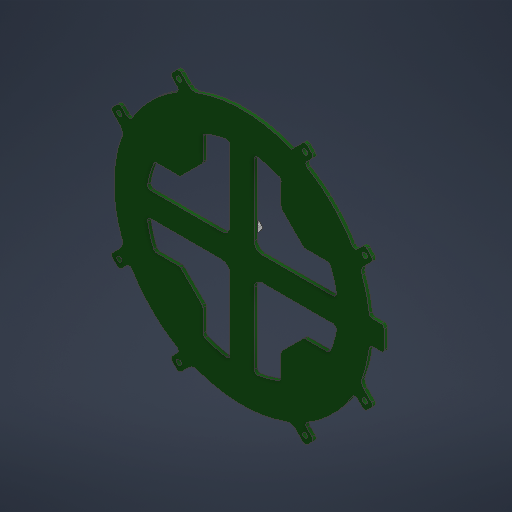
# Autodesk Inventor part: Line Board
Saved by Autodesk Inventor 2026.1 (Build 301233020, 233B)
## iProperties
Created: 2025-11-07
Part Number: Line Board
Material: Generic
Document SubType Name: Modeling
Designer: Bahaa
Density: 1 g/cm^3
Appearance: Default
Author: Bahaa
Autodesk Inventor part; units mm, degrees
ref_plane "YZ Plane" through (0, 0, 0) normal (1, 0, 0) x (0, 1, 0)
ref_plane "XZ Plane" through (0, 0, 0) normal (0, 1, 0) x (-1, 0, 0)
ref_plane "XY Plane" through (0, 0, 0) normal (0, 0, 1) x (1, 0, 0)
sketch "Sketch1" plane through (0, 0, 0) normal (0, 1, 0) x (-1, 0, 0)
  circle A0 centre (0, 0) radius 79
  circle A1 centre (0, 0) radius 59
  line L0 (-75, 7.5) -> (75, 7.5)
  line L1 (75, 7.5) -> (75, -7.5)
  line L2 (75, -7.5) -> (-75, -7.5)
  line L3 (-75, -7.5) -> (-75, 7.5)
  line L4 (-75, 7.5) -> (75, -7.5) construction
  line L5 (75, 7.5) -> (-75, -7.5) construction
  line L6 (-7.5, -75) -> (-7.5, 75)
  line L7 (7.5, 75) -> (7.5, -75)
  line L8 (75, -7.5) -> (-75, -7.5)
  line L9 (-75, 7.5) -> (75, 7.5)
  line L10 (7.5, 75) -> (7.5, -75)
  line L11 (-7.5, -75) -> (-7.5, 75)
  line L12 (7.5, 25) -> (-7.5, 25)
  line L13 (-25, 7.5) -> (-25, -7.5)
  line L14 (-7.5, -25) -> (7.5, -25)
  line L15 (25, -7.5) -> (25, 7.5)
  line L16 (25, 25) -> (-25, -25) construction
  line L17 (-25, 25) -> (25, -25) construction
  line L18 (-7.5, 25) -> (-25, 7.5)
  line L19 (25, 7.5) -> (7.5, 25)
  line L20 (25, -7.5) -> (7.5, -25)
  line L21 (-25, -7.5) -> (-7.5, -25)
  line L22 (0, 0) -> (57.2756, -57.2756) construction
  line L23 (57.2756, -57.2756) -> (38.8909, -75.6604) construction
  circle A2 centre (38.8909, -75.6604) radius 1.6
  line L24 (38.8909, -75.6604) -> (41.7193, -72.832) construction
  line L25 (41.7193, -72.832) -> (44.5477, -75.6604)
  line L26 (44.5477, -75.6604) -> (38.8909, -70.0036)
  line L27 (38.8909, -70.0036) -> (33.234, -75.6604) construction
  line L28 (33.234, -75.6604) -> (38.8909, -81.3173)
  line L29 (38.8909, -81.3173) -> (44.5477, -75.6604)
  line L30 (33.234, -75.6604) -> (30.4637, -72.8901)
  line L31 (38.8909, -70.0036) -> (38.0953, -69.208)
  circle A3 centre (75.6604, -38.8909) radius 1.6
  line L32 (75.6604, -38.8909) -> (72.832, -41.7193) construction
  line L33 (72.832, -41.7193) -> (75.6604, -44.5477)
  line L34 (75.6604, -44.5477) -> (70.0036, -38.8909)
  line L35 (70.0036, -38.8909) -> (75.6604, -33.234) construction
  line L36 (75.6604, -33.234) -> (81.3173, -38.8909)
  line L37 (81.3173, -38.8909) -> (75.6604, -44.5477)
  line L38 (75.6604, -33.234) -> (72.8901, -30.4637)
  line L39 (70.0036, -38.8909) -> (69.208, -38.0953)
  line L40 (70.0036, 38.8909) -> (69.208, 38.0953)
  line L41 (75.6604, 33.234) -> (72.8901, 30.4637)
  line L42 (70.0036, 38.8909) -> (75.6604, 33.234) construction
  line L43 (75.6604, 38.8909) -> (72.832, 41.7193) construction
  circle A4 centre (75.6604, 38.8909) radius 1.6
  line L44 (75.6604, 44.5477) -> (70.0036, 38.8909)
  line L45 (75.6604, 33.234) -> (81.3173, 38.8909)
  line L46 (81.3173, 38.8909) -> (75.6604, 44.5477)
  line L47 (57.2756, 57.2756) -> (75.6604, 38.8909) construction
  line L48 (72.832, 41.7193) -> (75.6604, 44.5477)
  line L49 (38.8909, 70.0036) -> (38.0953, 69.208)
  line L50 (41.7193, 72.832) -> (44.5477, 75.6604)
  line L51 (44.5477, 75.6604) -> (38.8909, 70.0036)
  line L52 (38.8909, 75.6604) -> (41.7193, 72.832) construction
  circle A5 centre (38.8909, 75.6604) radius 1.6
  line L53 (38.8909, 81.3173) -> (44.5477, 75.6604)
  line L54 (38.8909, 70.0036) -> (33.234, 75.6604) construction
  line L55 (33.234, 75.6604) -> (30.4637, 72.8901)
  line L56 (33.234, 75.6604) -> (38.8909, 81.3173)
  line L57 (-38.8909, 70.0036) -> (-38.0953, 69.208)
  line L58 (-33.234, 75.6604) -> (-30.4637, 72.8901)
  line L59 (-38.8909, 70.0036) -> (-33.234, 75.6604) construction
  line L60 (-38.8909, 75.6604) -> (-41.7193, 72.832) construction
  circle A6 centre (-38.8909, 75.6604) radius 1.6
  line L61 (-44.5477, 75.6604) -> (-38.8909, 70.0036)
  line L62 (-33.234, 75.6604) -> (-38.8909, 81.3173)
  line L63 (-38.8909, 81.3173) -> (-44.5477, 75.6604)
  line L64 (-57.2756, 57.2756) -> (-38.8909, 75.6604) construction
  line L65 (-41.7193, 72.832) -> (-44.5477, 75.6604)
  line L66 (-70.0036, 38.8909) -> (-69.208, 38.0953)
  line L67 (-72.832, 41.7193) -> (-75.6604, 44.5477)
  line L68 (-75.6604, 44.5477) -> (-70.0036, 38.8909)
  line L69 (-75.6604, 38.8909) -> (-72.832, 41.7193) construction
  circle A7 centre (-75.6604, 38.8909) radius 1.6
  line L70 (-81.3173, 38.8909) -> (-75.6604, 44.5477)
  line L71 (-70.0036, 38.8909) -> (-75.6604, 33.234) construction
  line L72 (-75.6604, 33.234) -> (-72.8901, 30.4637)
  line L73 (-75.6604, 33.234) -> (-81.3173, 38.8909)
  line L74 (-70.0036, -38.8909) -> (-69.208, -38.0953)
  line L75 (-75.6604, -33.234) -> (-72.8901, -30.4637)
  line L76 (-70.0036, -38.8909) -> (-75.6604, -33.234) construction
  line L77 (-75.6604, -38.8909) -> (-72.832, -41.7193) construction
  circle A8 centre (-75.6604, -38.8909) radius 1.6
  line L78 (-75.6604, -44.5477) -> (-70.0036, -38.8909)
  line L79 (-75.6604, -33.234) -> (-81.3173, -38.8909)
  line L80 (-81.3173, -38.8909) -> (-75.6604, -44.5477)
  line L81 (-57.2756, -57.2756) -> (-75.6604, -38.8909) construction
  line L82 (-72.832, -41.7193) -> (-75.6604, -44.5477)
  line L83 (-38.8909, -70.0036) -> (-38.0953, -69.208)
  line L84 (-41.7193, -72.832) -> (-44.5477, -75.6604)
  line L85 (-44.5477, -75.6604) -> (-38.8909, -70.0036)
  line L86 (-38.8909, -75.6604) -> (-41.7193, -72.832) construction
  circle A9 centre (-38.8909, -75.6604) radius 1.6
  line L87 (-38.8909, -81.3173) -> (-44.5477, -75.6604)
  line L88 (-38.8909, -70.0036) -> (-33.234, -75.6604) construction
  line L89 (-33.234, -75.6604) -> (-30.4637, -72.8901)
  line L90 (-33.234, -75.6604) -> (-38.8909, -81.3173)
  line L91 (55.8614, 55.8614) -> (71.4178, 40.3051) construction
  line L92 (71.4178, 40.3051) -> (71.3471, 40.2344) construction
  line L93 (71.3471, 40.2344) -> (40.2344, 71.3471)
  line L94 (-40.2344, 71.3471) -> (-71.3471, 40.2344)
  line L95 (-71.3471, -40.2344) -> (-40.2344, -71.3471)
  line L96 (40.2344, -71.3471) -> (71.3471, -40.2344)
  line L97 (70.25, -7.5) -> (87.75, -7.5)
  line L98 (87.75, -7.5) -> (87.75, 7.5)
  line L99 (87.75, 7.5) -> (70.25, 7.5)
  line L100 (70.25, 7.5) -> (70.25, -7.5)
  line L101 (70.25, -7.5) -> (87.75, 7.5) construction
  line L102 (87.75, -7.5) -> (70.25, 7.5) construction
  line L103 (0, -7.5) -> (0, 7.5) construction
  line L104 (-70.25, -7.5) -> (-87.75, -7.5)
  line L105 (-87.75, -7.5) -> (-87.75, 7.5)
  line L106 (-87.75, 7.5) -> (-70.25, 7.5)
  line L107 (-70.25, 7.5) -> (-70.25, -7.5)
  line L108 (10, 44) -> (-10, 44)
  line L109 (-10, 44) -> (-10, 59) construction
  line L110 (-10, 59) -> (10, 59) construction
  line L111 (10, 59) -> (10, 44) construction
  line L112 (10, 44) -> (-10, 59) construction
  line L113 (-10, 44) -> (10, 59) construction
  line L114 (10, 44) -> (21.0986, 55.0986)
  line L115 (10, 44) -> (24.951, 44) construction
  line L116 (-10, 44) -> (-21.0986, 55.0986)
  line L117 (-38.1838, 24.0416) -> (-53.8795, 24.0416)
  line L118 (-24.0416, 38.1838) -> (-38.1838, 24.0416)
  line L119 (-24.0416, 38.1838) -> (-24.0416, 53.8795)
  line L120 (-44, -10) -> (-55.0986, -21.0986)
  line L121 (-44, 10) -> (-44, -10)
  line L122 (-44, 10) -> (-55.0986, 21.0986)
  line L123 (-24.0416, -38.1838) -> (-24.0416, -53.8795)
  line L124 (-38.1838, -24.0416) -> (-24.0416, -38.1838)
  line L125 (-38.1838, -24.0416) -> (-53.8795, -24.0416)
  line L126 (10, -44) -> (21.0986, -55.0986)
  line L127 (-10, -44) -> (10, -44)
  line L128 (-10, -44) -> (-21.0986, -55.0986)
  line L129 (38.1838, -24.0416) -> (53.8795, -24.0416)
  line L130 (24.0416, -38.1838) -> (38.1838, -24.0416)
  line L131 (24.0416, -38.1838) -> (24.0416, -53.8795)
  line L132 (44, 10) -> (55.0986, 21.0986)
  line L133 (44, -10) -> (44, 10)
  line L134 (44, -10) -> (55.0986, -21.0986)
  line L135 (24.0416, 38.1838) -> (24.0416, 53.8795)
  line L136 (38.1838, 24.0416) -> (24.0416, 38.1838)
  line L137 (38.1838, 24.0416) -> (53.8795, 24.0416)
  point P0 (-58.5214, 7.5)
  point P1 (-7.5, 58.5214)
  point P2 (-7.5, 25)
  point P3 (-25, 7.5)
  point P4 (-58.5214, -7.5)
  point P5 (-25, -7.5)
  point P6 (-7.5, -25)
  point P7 (-7.5, -58.5214)
  point P8 (-74.6241, 7.5)
  point P9 (-74.6241, -7.5)
  point P10 (-72.8901, -30.4637)
  point P11 (-30.4637, -72.8901)
  point P12 (69.208, -38.0953)
  point P13 (72.8901, -30.4637)
  point P14 (74.6241, -7.5)
  point P15 (74.6241, 7.5)
  point P16 (72.8901, 30.4637)
  point P17 (69.208, 38.0953)
  point P18 (38.0953, 69.208)
  point P19 (30.4637, 72.8901)
  point P20 (-38.0953, 69.208)
  point P21 (-69.208, 38.0953)
  point P22 (-72.8901, 30.4637)
  point P23 (58.5214, -7.5)
  point P24 (7.5, -58.5214)
  point P25 (7.5, -25)
  point P26 (25, -7.5)
  point P27 (58.5214, 7.5)
  point P28 (25, 7.5)
  point P29 (7.5, 25)
  point P30 (7.5, 58.5214)
  point P31 (-38.8202, 69.9329)
  point P32 (-69.9329, 38.8202)
  point P33 (-69.9329, -38.8202)
  point P34 (-38.8202, -69.9329)
  point P35 (38.8202, -69.9329)
  point P36 (69.9329, -38.8202)
  point P37 (-71.3471, -40.2344)
  point P38 (-58.6005, -52.9809)
  point P39 (-40.2344, -71.3471)
  point P40 (-52.9809, -58.6005)
  point P41 (-52.9809, 58.6005)
  point P42 (40.2344, -71.3471)
  point P43 (52.9809, -58.6005)
  point P44 (58.6005, -52.9809)
  point P45 (58.6005, 52.9809)
  point P46 (52.9809, 58.6005)
  point P47 (-58.6005, 52.9809)
  point P48 (-71.3471, 40.2344)
  point P49 (79, 0)
  point P50 (78.6432, 7.5)
  point P51 (78.6432, -7.5)
  point P52 (-78.6432, -7.5)
  point P53 (-78.6432, 7.5)
  point P54 (0, 0)
  point P55 (-7.5, 7.5)
  point P56 (-7.5, -7.5)
  point P57 (7.5, -7.5)
  point P58 (7.5, 7.5)
  point P59 (0, 51.5)
  dimension "d0" = 158
  dimension "d1" = 20
  dimension "d2" = 150
  dimension "d3" = 15
  dimension "d6" = 360
  dimension "d8" = 50
  dimension "d9" = 50
  dimension "d10" = 17.5
  dimension "d11" = 17.5
  dimension "d12" = 17.5
  dimension "d13" = 17.5
  dimension "d14" = 17.5
  dimension "d15" = 17.5
  dimension "d16" = 17.5
  dimension "d17" = 17.5
  dimension "d18" = 81
  dimension "d19" = 26
  dimension "d20" = 3.2
  dimension "d23" = 4
  dimension "d24" = 4
  dimension "d25" = 8
  dimension "d26" = 8
  dimension "d27" = 8
  dimension "d30" = 360
  dimension "d36" = 0.1
  dimension "d39" = 360
  dimension "d50" = 17.5
  dimension "d51" = 15
  dimension "d52" = 70.25
  dimension "d68" = 15
  dimension "d69" = 20
  dimension "d70" = 0
  dimension "d71" = 0
  dimension "d73" = 45
  dimension "d76" = 360
  constraints: 276 end point, 23 point on line, 14 symmetric about line, 11 midpoint, 10 parallel, 10 perpendicular, 9 coincident, 8 centre point, 5 horizontal, 259 other
  measures "d2" distance of L1.end L2.end
  measures "d3" distance of L0.end L1.end
  measures "d8" distance of L17.end L16.end
  measures "d9" distance of L16.end L17.start
  measures "d10" distance of L12.end L17.start
  measures "d11" distance of L13.start L17.start
  measures "d12" distance of L15.end L16.start
  measures "d13" distance of L12.start L16.start
  measures "d14" distance of L15.start L17.end
  measures "d15" distance of L14.end L17.end
  measures "d16" distance of L13.end L16.end
  measures "d17" distance of L14.start L16.end
  measures "d18" distance of L22.start L22.end
  measures "d19" distance of L22.end L23.end
  measures "d20" diameter of A2
  measures "d23" distance of L24.start L24.end
  measures "d24" distance of L24.end L25.end
  measures "d25" distance of L25.end L26.end
  measures "d26" distance of L27.end L26.end
  measures "d27" distance between parallel lines of L30 L31
  measures "d36" distance of L91.end L92.end
  measures "d50" distance of L99.end L98.end
  measures "d51" distance of L98.end L97.end
  measures "d52" distance from line of L22.start L100
  measures "d68" distance of L108.end L109.end
  measures "d69" distance of L108.start L108.end
  measures "d70" vertical extent of L110
  measures "d71" horizontal distance of L22.start point (0, 51.5)
  measures "d73" angle of L115 L114
extrude "Extrusion1" add sketch "Sketch1" along normal blind 2 contours A0 L99 L0 A1 L106 L94 L93 | A0 L40 L44 L46 L45 L41 | A0 L97 L1 L99 | L1 L2 L100 L0 | A0 L96 L95 L104 L2 A1 L97 | L100 L2 A1 L0 | A0 L55 L56 L53 L50 L51 L49 | L38 L36 L37 L33 L34 L39 A0 | A1 L2 L133 L0 | L133 L2 L15 L0 | A0 L57 L61 L63 L62 L58 | L137 L136 L135 A1 | L15 L2 L7 L0 | L7 L2 L6 L0 | L0 L6 L12 L7 | L12 L6 L108 L7 | A1 L131 L130 L129 | L31 L26 L25 L29 L28 L30 A0 | L6 L2 L13 L0 | L7 L14 L6 L2 | L7 L127 L6 L14 | L108 L6 A1 L7 | L13 L2 L121 L0 | L7 A1 L6 L127 | A0 L72 L73 L70 L67 L68 L66 | L89 L90 L87 L84 L85 L83 A0 | L121 L2 A1 L0 | A1 L2 L107 L0 | L106 L3 L104 A0 | A0 L104 L105 L106 | L119 L118 L117 A1 | L107 L2 L3 L0 | A1 L125 L124 L123 | A0 L74 L78 L80 L79 L75
fillet "Fillet1" radius 2 52 edges at (-81.3173, 1, 38.8909) (-75.6604, 1, 44.5477) (-38.8909, 1, 81.3173) (-44.5477, 1, 75.6604) (38.8909, 1, 81.3173) (44.5477, 1, 75.6604) (75.6604, 1, 44.5477) (81.3173, 1, 38.8909) (81.3173, 1, -38.8909) (75.6604, 1, -44.5477) (44.5477, 1, -75.6604) (38.8909, 1, -81.3173) (-44.5477, 1, -75.6604) (-38.8909, 1, -81.3173) (-81.3173, 1, -38.8909) (-75.6604, 1, -44.5477) (-7.5, 1, 58.5214) (-58.5214, 1, 7.5) (-58.5214, 1, -7.5) (-7.5, 1, -58.5214) (7.5, 1, -58.5214) (58.5214, 1, -7.5) (58.5214, 1, 7.5) (7.5, 1, 58.5214) (69.208, 1, -38.0953) (38.0953, 1, -69.208) (-38.0953, 1, -69.208) (-69.208, 1, -38.0953) (-69.208, 1, 38.0953) (-38.0953, 1, 69.208) (38.0953, 1, 69.208) (69.208, 1, 38.0953) (78.6432, 1, -7.5) (87.75, 1, -7.5) (87.75, 1, 7.5) (78.6432, 1, 7.5) (24.0416, 1, 38.1838) (24.0416, 1, 53.8795) (38.1838, 1, 24.0416) (53.8795, 1, 24.0416) (53.8795, 1, -24.0416) (38.1838, 1, -24.0416) (24.0416, 1, -38.1838) (24.0416, 1, -53.8795) (-24.0416, 1, -53.8795) (-24.0416, 1, -38.1838) (-38.1838, 1, -24.0416) (-53.8795, 1, -24.0416) (-53.8795, 1, 24.0416) (-38.1838, 1, 24.0416) (-24.0416, 1, 38.1838) (-24.0416, 1, 53.8795)
fillet "Fillet2" radius 5 11 edges at (72.8901, 1, 30.4637) (72.8901, 1, -30.4637) (30.4637, 1, -72.8901) (-30.4637, 1, -72.8901) (-72.8901, 1, -30.4637) (-72.8901, 1, 30.4637) (-30.4637, 1, 72.8901) (7.5, 1, -7.5) (7.5, 1, 7.5) (-7.5, 1, 7.5) (-7.5, 1, -7.5)
sketch "Sketch2" plane through (0, 2, 0) normal (0, -1, 0) x (1, 0, 0)
  line L0 (-65, -15) -> (65, -15) construction
  line L1 (65, -15) -> (65, 15) construction
  line L2 (65, 15) -> (-65, 15) construction
  line L3 (-65, 15) -> (-65, -15) construction
  line L4 (-65, -15) -> (65, 15) construction
  line L5 (65, -15) -> (-65, 15) construction
  line L6 (0, 15) -> (0, 12) construction
  line L7 (0, 0) -> (65, 0) construction
  circle A0 centre (0, 12) radius 1.35
  circle A1 centre (0, 12) radius 2.55
  circle A2 centre (0, -12) radius 1.35
  circle A3 centre (0, -12) radius 2.55
  dimension "d41" = 130
  dimension "d42" = 30
  dimension "d43" = 3
  dimension "d44" = 2.7
  dimension "d45" = 5.1
  dimension "d46" = 2.7
  dimension "d47" = 5.1
  constraints: 16 end point, 5 coincident, 4 centre point, 4 midpoint, 2 parallel, 1 horizontal, 1 perpendicular, 1 symmetric about line, 1 vertical
  measures "d41" distance of L2.end L1.end
  measures "d42" distance of L1.end L0.end
  measures "d43" distance of L6.start L6.end
  measures "d44" diameter of A0
  measures "d45" diameter of A1
  measures "d46" diameter of A2
  measures "d47" diameter of A3
extrude "Extrusion2" add sketch "Sketch2" against normal blind 8 from surface at 0
equation "\"d11\" = d10"
equation "\"d12\" = d10"
equation "\"d13\" = d12"
equation "\"d14\" = d10"
equation "\"d15\" = d14"
equation "\"d16\" = d10"
equation "\"d17\" = d16"
equation "\"d24\" = d23"
equation "\"d25\" = 2 * d23"
equation "\"d27\" = 2 * d23"
body "Solid1"
